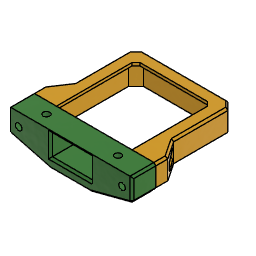
cnc3018_Z-Energie_Holder v5 (Autodesk Fusion 360 design; units mm, degrees)
Autodesk Fusion 360 part; units mm, degrees
sketch "Skizze1" plane through (0, 0, 0) normal (0, 0, 1) x (1, 0, 0) in component "StepperBügel"
  line L0 (0, 0) -> (0, 42)
  line L1 (0, 42) -> (42, 42)
  line L2 (42, 42) -> (42, 0)
  line L3 (42, 0) -> (46, 0)
  line L4 (46, 0) -> (46, 46)
  line L5 (46, 46) -> (-4, 46)
  line L6 (-4, 46) -> (-4, 0)
  line L7 (-4, 0) -> (0, 0)
  line L8 (-4, 0) -> (-10, 0)
  line L9 (-10, 0) -> (-10, 6)
  line L10 (-10, 6) -> (-4, 15)
  line L11 (21, 46) -> (21, 0)
  line L12 (46, 0) -> (52, 0)
  line L13 (52, 0) -> (52, 6)
  line L14 (52, 6) -> (46, 15)
  dimension "d1" = 4
  dimension "d2" = 4
  dimension "d3" = 42
  dimension "d4" = 42
  dimension "d5" = 10
  dimension "d6" = 6
  dimension "d7" = 15
  constraint coincident L0.start L7.end
  constraint vertical L0
  constraint perpendicular L0 L1
  constraint perpendicular L1 L2
  constraint perpendicular L2 L3
  constraint perpendicular L3 L4
  constraint perpendicular L4 L5
  constraint perpendicular L5 L6
  constraint perpendicular L6 L7
  constraint equal L3 L7
  constraint collinear L3 L7
  constraint perpendicular L6 L8
  constraint perpendicular L8 L9
  constraint coincident L6 L10.end
  constraint midpoint L5 L11.start
  constraint perpendicular L5 L11
  constraint symmetric L6.end L11 L3.end
  constraint symmetric L8.end L11 L12.end
  constraint symmetric L9.end L11 L13.end
  constraint symmetric L10.end L11 L14.end
  measures "d1" distance of L6.end L0.start
  measures "d2" distance of L1 L5
  measures "d3" distance of L0 L2
  measures "d4" distance of L1 L7
  measures "d5" distance of L0 L9
  measures "d6" distance of L8.end L9.end
  measures "d7" distance of L8 L10.end
extrude "Extrusion1" add sketch "Skizze1" along normal blind 10 makes body 1 in component "StepperBügel"
sketch "Skizze2" plane through (0, 0, 0) normal (0, -1, 0) x (1, 0, 0) in component "StepperBügel"
  line L0 (-10, 0) -> (0, 0)
  line L1 (0, 0) -> (0, 10)
  line L2 (0, 10) -> (-10, 10)
  line L3 (-10, 10) -> (-10, 0)
  line L4 (-5, 0) -> (-5, 5)
  line L5 (-5, 5) -> (-10, 5)
  circle A0 centre (-5, 5) radius 1.65
  line L6 (-2.1, 6.6743) -> (-5, 8.3486)
  line L7 (-5, 8.3486) -> (-7.9, 6.6743)
  line L8 (-7.9, 6.6743) -> (-7.9, 3.3257)
  line L9 (-7.9, 3.3257) -> (-5, 1.6514)
  line L10 (-5, 1.6514) -> (-2.1, 3.3257)
  line L11 (-2.1, 3.3257) -> (-2.1, 6.6743)
  point P0 (-5, 5)
  dimension "d10" = 3.3
  dimension "d12" = 5.8
  constraint midpoint L0 L4.start
  constraint perpendicular L0 L4
  constraint midpoint L3 L5.end
  constraint perpendicular L3 L5
  constraint coincident P0 L4.end
  measures "d10" diameter of A0
  measures "d12" distance of L8 L11
extrude "Extrusion2" cut sketch "Skizze2" against normal blind 15 contours L4 L5 A0 | L4 L5 A0 bodies 1 in component "StepperBügel"
extrude "Extrusion3" cut sketch "Skizze2" against normal blind 12 from surface at -3 contours L4 L5 A0 L8 L9 | L4 L5 A0 L6 L7 L8 L10 L11 bodies 1 in component "StepperBügel"
chamfer "Fase1" distance 0.5 angle 45 5 edges at (-4.5, 14.25, 8.06) (-6.45, 11.325, 7.5115) (-7.9, 9.15, 5) (-6.45, 11.325, 2.4885) (-4.5, 14.25, 1.94) on bodies 1 in component "StepperBügel"
ref_plane "Arbeitsebene1" through (21, 21, 5) normal (1, 0, 0) x (0, 1, 0) in component "StepperBügel"
mirror "Spiegeln1" about plane through (21, 21, 5) normal (1, 0, 0) of "Extrusion2", "Extrusion3", "Fase1" in component "StepperBügel"
sketch "Skizze3" plane through (0, 0, 10) normal (0, 0, 1) x (-1, 0, 0) in component "StepperBügel"
  line L0 (10, 0) -> (0, 0)
  line L1 (0, 0) -> (0, -42)
  line L2 (0, -42) -> (-42, -42)
  line L3 (-42, -42) -> (-42, 0)
  line L4 (-42, 0) -> (-52, 0)
  line L5 (-52, 0) -> (-52, -6)
  line L6 (-52, -6) -> (-46, -15)
  line L7 (-46, -15) -> (-46, -46)
  line L8 (-46, -46) -> (4, -46)
  line L9 (4, -46) -> (4, -15)
  line L10 (4, -15) -> (10, -6)
  line L11 (10, -6) -> (10, 0)
  line L12 (0, 0) -> (-2, 0)
  line L13 (-2, 0) -> (-2, -40)
  line L14 (-2, -40) -> (-40, -40)
  line L15 (-40, -40) -> (-40, 0)
  line L16 (-40, 0) -> (-42, 0)
  line L17 (-42, 0) -> (-42, -42)
  line L18 (-42, -42) -> (0, -42)
  line L19 (0, -42) -> (0, 0)
  dimension "d21" = 2
  dimension "d22" = 2
  dimension "d23" = 2
  constraint coincident L0.end L1.start
  constraint perpendicular L1 L12
  constraint perpendicular L0 L13
  constraint perpendicular L1 L14
  constraint perpendicular L14 L15
  constraint coincident L3.end L4.start
  constraint perpendicular L3 L16
  constraint coincident L2.end L3.start
  constraint coincident L1.end L2.start
  measures "d21" distance of L13 L19
  measures "d22" distance of L14 L18
  measures "d23" distance of L15 L17
extrude "Extrusion4" add sketch "Skizze3" along normal blind 1.5 bodies 1 in component "StepperBügel"
chamfer "Fase2" distance 2 angle 45 2 edges at (2, 40, 10.75) (40, 40, 10.75) on bodies 1 in component "StepperBügel"
chamfer "Fase2" distance 3.8 angle 45 4 edges at (0, 42, 5) (42, 42, 5) (46, 46, 5.75) (-4, 46, 5.75) on bodies 1 in component "StepperBügel"
chamfer "Fase2" distance 1 angle 45 14 edges at (52, 3, 11.5) (49, 10.5, 11.5) (46, 30.5, 11.5) (21, 46, 11.5) (-4, 30.5, 11.5) (-7, 10.5, 11.5) (-10, 3, 11.5) (-10, 3, 0) (-7, 10.5, 0) (-4, 30.5, 0) (21, 46, 0) (46, 30.5, 0) (49, 10.5, 0) (52, 3, 0) on bodies 1 in component "StepperBügel"
sketch "Skizze1 (2)" plane through (0, 0, 0) normal (0, -1, 0) x (1, 0, 0) in component "StepperVerschluss"
  circle A0 centre (-5, 5) radius 1.65
  line L0 (-9, 11.5) -> (-10, 10.5)
  line L1 (-10, 10.5) -> (-10, 1)
  line L2 (-10, 1) -> (-9, 0)
  line L3 (-9, 0) -> (0, 0)
  line L4 (0, 0) -> (0, 10)
  line L5 (0, 10) -> (2, 10)
  line L6 (2, 10) -> (2, 11.5)
  line L7 (2, 11.5) -> (-9, 11.5)
  line L8 (-10, 11.5) -> (52, 11.5)
  line L9 (52, 0) -> (-10, 0)
  line L10 (-10, 11.5) -> (-10, 0)
  line L11 (52, 11.5) -> (52, 0)
  circle A1 centre (47, 5) radius 1.65
  circle A2 centre (-5, 5) radius 1.65
  line L12 (21, 11.5) -> (21, 0) construction
  line L13 (21, 10) -> (11, 10)
  line L14 (11, 10) -> (11, -0.5)
  line L15 (11, -0.5) -> (21, -0.5)
  line L16 (21, 10) -> (31, 10)
  line L17 (31, 10) -> (31, -0.5)
  line L18 (31, -0.5) -> (21, -0.5)
  line L19 (21, -5.5) -> (11, -5.5)
  line L20 (11, -5.5) -> (-10, 0)
  line L21 (31, -5.5) -> (52, 0)
  line L22 (21, -5.5) -> (31, -5.5)
  dimension "d29" = 62
  dimension "d30" = 11.5
  dimension "d31" = 10
  dimension "d34" = 20
  dimension "d35" = 1.5
  dimension "d36" = 12
  dimension "d37" = 5
  dimension "d38" = 20
  constraint perpendicular L6 L8
  constraint perpendicular L1 L9
  constraint vertical L11
  constraint coincident L3.end L9
  constraint midpoint L8 L12.start
  constraint midpoint L9 L12.end
  constraint coincident L12 L13.start
  constraint perpendicular L12 L13
  constraint perpendicular L9 L14
  constraint perpendicular L14 L15
  constraint symmetric L12 L13.start L16.start
  constraint symmetric L12 L13.end L16.end
  constraint symmetric L12 L14.end L17.end
  constraint symmetric L12 L15.end L18.end
  constraint perpendicular L4 L19
  constraint coincident L12 L19.start
  constraint symmetric L9.end L12 L9.start
  constraint symmetric L12 L19.start L22.start
  constraint symmetric L12 L19.end L21.start
  measures "d29" distance of L10 L11
  measures "d30" distance of L8 L9
  measures "d31" distance of L3.end L10
  measures "d34" distance of L14 L17
  measures "d35" distance of L8 L13
  measures "d36" distance of L8 L15
  measures "d37" distance of L15 L19
  measures "d38" distance of L19.end L21.start
extrude "Extrusion1'" add sketch "Skizze1 (2)" along normal blind 12 separate body contours L0 L1 L2 L3 L4 L5 L6 L7 L8 L9 L10 | L0 L8 L10 | L4 L5 L6 L8 L9 L11 L13 L14 L16 L17 | L2 L9 L10 | L3 L9 L14 L15 L17 L18 L19 L20 L21 L22 makes body 2 in component "StepperVerschluss"
chamfer "Fase1'" distance 1 angle 45 8 edges at (21, -12, 10) (31, -12, 4.75) (21, -12, -0.5) (11, -12, 4.75) (-10, -6, 11.5) (-10, -6, 0) (52, -6, 0) (52, -6, 11.5) on bodies 2 in component "StepperVerschluss"
chamfer "Fase1'" distance 1 angle 45 5 edges at (-10, -12, 5.75) (0.5, -12, -2.75) (21, -12, -5.5) (41.5, -12, -2.75) (52, -12, 5.75) on bodies 2 in component "StepperVerschluss"
sketch "Skizze2 (2)" plane through (0, 0, 11.5) normal (0, 0, 1) x (-1, 0, 0) in component "StepperVerschluss"
  line L0 (-51, 12) -> (-51, 0)
  line L1 (-51, 0) -> (9, 0)
  line L2 (9, 0) -> (9, 12)
  line L3 (9, 12) -> (-51, 12)
  line L4 (-11, 0) -> (-11, 11)
  line L5 (-21, 0) -> (-21, 12)
  circle A0 centre (-3, 6) radius 1.65
  circle A1 centre (-39, 6) radius 1.65
  line L6 (9, 6) -> (-3, 6) construction
  line L7 (-4.6743, 8.9) -> (-6.3486, 6)
  line L8 (-6.3486, 6) -> (-4.6743, 3.1)
  line L9 (-4.6743, 3.1) -> (-1.3257, 3.1)
  line L10 (-1.3257, 3.1) -> (0.3486, 6)
  line L11 (0.3486, 6) -> (-1.3257, 8.9)
  line L12 (-1.3257, 8.9) -> (-4.6743, 8.9)
  line L13 (-40.6743, 3.1) -> (-42.3486, 6)
  line L14 (-42.3486, 6) -> (-40.6743, 8.9)
  line L15 (-40.6743, 8.9) -> (-37.3257, 8.9)
  line L16 (-37.3257, 8.9) -> (-35.6514, 6)
  line L17 (-37.3257, 3.1) -> (-40.6743, 3.1)
  line L18 (-35.6514, 6) -> (-37.3257, 3.1)
  point P0 (-3, 6)
  dimension "d41" = 3.3
  dimension "d42" = 36
  dimension "d43" = 5.8
  constraint midpoint L1 L5.start
  constraint midpoint L3 L5.end
  constraint symmetric L5 A0 A1
  constraint midpoint L2 L6.start
  constraint coincident P0 A0.centre
  constraint perpendicular L2 L6
  constraint symmetric L5 L7.start L15.end
  constraint symmetric L5 L7.end L16.end
  constraint symmetric L5 L8.end L17.start
  constraint symmetric L5 L9.end L13.start
  constraint symmetric L5 L10.end L13.end
  constraint symmetric L5 L11.end L14.end
  measures "d41" diameter of A0
  measures "d42" distance of P0 A1.centre
  measures "d43" distance of L9 L12
extrude "Extrusion2'" cut sketch "Skizze2 (2)" against normal through all contours A0 | A1 bodies 2 in component "StepperVerschluss"
extrude "Extrusion3'" cut sketch "Skizze2 (2)" against normal through all from surface at -3 contours L7 L8 L9 L10 L11 L12 | L13 L14 L15 L16 L17 L18 bodies 2 in component "StepperVerschluss"
component "StepperBügel" placed x (1, 0, 0) y (0, 1, 0) z (0, 0, 1) at (0, 0, 0)
component "StepperVerschluss" placed x (1, 0, 0) y (0, 1, 0) z (0, 0, 1) at (0, 0, 0)
